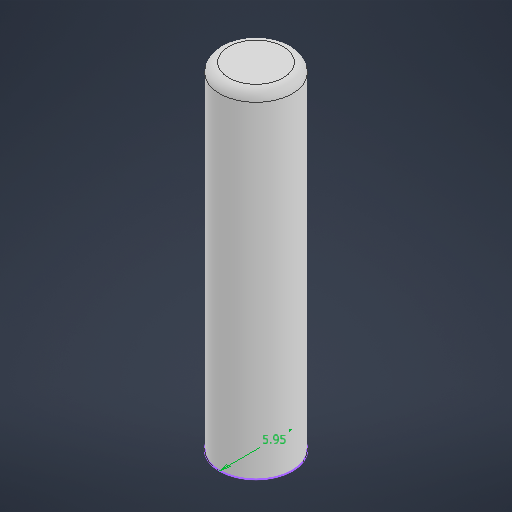
# Autodesk Inventor part: ControllerButton
Saved by Autodesk Inventor 2026.2 (Build 302298010, 298A)
## iProperties
Created: 2026-06-02
Part Number: ControllerButton
Material: Generic
Document SubType Name: Modeling
Designer: barbe
Density: 1 g/cm^3
Appearance: Default
Author: barbe
Autodesk Inventor part; units mm, degrees
ref_plane "YZ Plane" through (0, 0, 0) normal (1, 0, 0) x (0, 1, 0)
ref_plane "XZ Plane" through (0, 0, 0) normal (0, 1, 0) x (-1, 0, 0)
ref_plane "XY Plane" through (0, 0, 0) normal (0, 0, 1) x (1, 0, 0)
sketch "Sketch1" plane through (0, 0, 0) normal (0, 1, 0) x (-1, 0, 0)
  circle A0 centre (0, 0) radius 2.975
  dimension "d1" = 5.95
  constraints: 1 centre point
  measures "d1" diameter of A0
extrude "Extrusion4" add sketch "Sketch1" along normal blind 27.5
fillet "Fillet3" radius 0.75 1 edges at (2.975, 27.5, 0)
body "Solid2"
